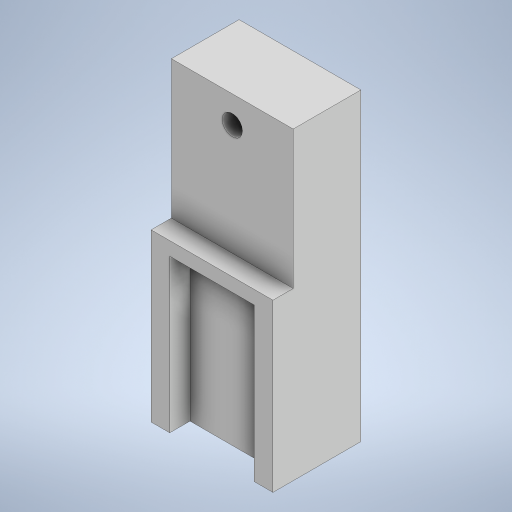
# Autodesk Inventor part: ジョイントモーター付き
Saved by Autodesk Inventor 2023 (Build 270158000, 158)
## iProperties
Created: 2023-10-21
Part Number: ジョイントモーター付き
Material: 一般
Document SubType Name: Modeling
Designer: ukkun
Density: 1 g/cm^3
Appearance: 既定
Author: ukkun
Autodesk Inventor part; units mm, degrees
ref_plane "YZ Plane" through (0, 0, 0) normal (1, 0, 0) x (0, 1, 0)
ref_plane "XZ Plane" through (0, 0, 0) normal (0, 1, 0) x (-1, 0, 0)
ref_plane "XY Plane" through (0, 0, 0) normal (0, 0, 1) x (1, 0, 0)
sketch "スケッチ1" plane through (0, 0, 0) normal (0, 0, 1) x (1, 0, 0)
  line L0 (-9, -22.5) -> (9, -22.5)
  line L1 (9, -22.5) -> (9, 22.5)
  line L2 (9, 22.5) -> (-9, 22.5)
  line L3 (-9, 22.5) -> (-9, -22.5)
  line L4 (-9, -22.5) -> (9, 22.5) construction
  line L5 (9, -22.5) -> (-9, 22.5) construction
  point P0 (0, 0)
  dimension "d0" = 18
  dimension "d1" = 45
  constraints: 12 end point, 2 midpoint, 2 parallel, 1 horizontal, 1 perpendicular
  measures "d0" distance of L1.end L2.end
  measures "d1" distance of L2.end L0.start
extrude "押し出し1" add sketch "スケッチ1" along normal blind 10
sketch "スケッチ2" plane through (0, 0, 10) normal (0, 0, 1) x (1, 0, 0)
  line L0 (-9, 22.5) -> (-9, -22.5) projected
  line L1 (-9, -22.5) -> (-9, 2.1)
  line L2 (-9, 2.1) -> (9, 2.1)
  line L3 (9, -22.5) -> (9, 22.5) projected
  line L4 (9, 2.1) -> (9, -22.5)
  line L5 (9, -22.5) -> (6.25, -22.5)
  line L6 (-9, -22.5) -> (9, -22.5) projected
  line L7 (6.25, -22.5) -> (6.25, 0.1)
  line L8 (6.25, 0.1) -> (-6.25, 0.1)
  line L9 (-6.25, 0.1) -> (-6.25, -22.5)
  line L10 (-9, -22.5) -> (-6.25, -22.5)
  point P0 (0, 0)
  dimension "d4" = 12.5
  dimension "d5" = 2.75
  dimension "d6" = 22.6
  dimension "d7" = 2
  constraints: 16 end point, 4 point on line, 3 perpendicular, 2 collinear, 1 vertical
  measures "d4" distance between parallel lines of L7 L9
  measures "d5" distance between parallel lines of L3 L7
  measures "d6" distance of L5.end L7.end
  measures "d7" distance between parallel lines of L2 L8
extrude "押し出し2" add sketch "スケッチ2" along normal blind 3 contours L2 L3 L5 L7 L8 L9 L6 L0
sketch "スケッチ3" plane through (0, 0, 10) normal (0, 0, 1) x (1, 0, 0)
  circle A0 centre (0, 18.5) radius 1.5
  line L0 (9, 22.5) -> (-9, 22.5) projected
  point P0 (0, 0)
  dimension "d10" = 3
  dimension "d11" = 4
  constraints: 1 centre point
  measures "d10" diameter of A0
  measures "d11" distance from line of L0 A0.centre
extrude "押し出し3" cut sketch "スケッチ3" against normal through all
sketch "スケッチ4" plane through (-9, -22.5, 0) normal (0, -1, 0) x (1, 0, 0)
  circle A0 centre (9, 5) radius 1.5
  line L0 (18, 0) -> (18, 13) projected
  line L1 (0, 0) -> (18, 0) projected
  point P0 (9, 0)
  dimension "d14" = 3
  dimension "d15" = 9
  dimension "d16" = 5
  constraints: 1 centre point
  measures "d14" diameter of A0
  measures "d15" distance from line of L0 A0.centre
  measures "d16" distance from line of L1 A0.centre
extrude "押し出し4" cut sketch "スケッチ4" against normal blind 25
